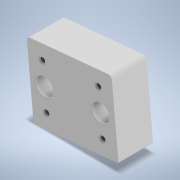
# Autodesk Inventor part: Head Spacer Plate
Saved by Autodesk Inventor 2020 (Build 240168000, 168)
## iProperties
Created: 2020-03-19
Part Number: Head Spacer Plate
Material: Generic
Document SubType Name: Modeling
Designer: DasNick
Density: 1 g/cm^3
Appearance: Default
Author: DasNick
Autodesk Inventor part; units mm, degrees
ref_plane "YZ Plane" through (0, 0, 0) normal (1, 0, 0) x (0, 1, 0)
ref_plane "XZ Plane" through (0, 0, 0) normal (0, 1, 0) x (-1, 0, 0)
ref_plane "XY Plane" through (0, 0, 0) normal (0, 0, 1) x (1, 0, 0)
sketch "Sketch1" plane through (0, 0, 0) normal (0, 0, 1) x (1, 0, 0)
  arc A0 (17.6188, 35.9553) -> (15.4359, 37.7539) centre (15.6281, 35.7632) ccw projected
  line L0 (15.4359, 37.7539) -> (-27.3652, 33.6227) projected
  arc A1 (-27.3652, 33.6227) -> (-29.1638, 31.4398) centre (-27.173, 31.6319) ccw projected
  line L1 (-29.1638, 31.4398) -> (-25.5552, -5.9466) projected
  arc A2 (-25.5552, -5.9466) -> (-25.0095, -6.3962) centre (-25.0575, -5.8985) ccw projected
  line L2 (-25.0095, -6.3962) -> (20.7777, -1.9768) projected
  arc A3 (20.7777, -1.9768) -> (21.2274, -1.4311) centre (20.7297, -1.4791) ccw projected
  line L3 (21.2274, -1.4311) -> (17.6188, 35.9553) projected
  circle A4 centre (-19.4703, 14.2799) radius 4.75 projected
  circle A5 centre (11.3863, 17.2582) radius 4.75 projected
  circle A6 centre (-18.3261, 2.3283) radius 1.25 projected
  circle A7 centre (10.2334, 29.2027) radius 1.25 projected
  circle A8 centre (-20.6232, 26.2244) radius 1.25 projected
  circle A9 centre (12.5491, 5.3084) radius 1.25 projected
  circle A10 centre (-18.3261, 2.3283) radius 1.5
  circle A11 centre (12.5491, 5.3084) radius 1.5
  circle A12 centre (10.2334, 29.2027) radius 1.5
  circle A13 centre (-20.6232, 26.2244) radius 1.5
  point P0 (0, 0)
  dimension "d0" = 3
  dimension "d1" = 3
  dimension "d3" = 3
  dimension "d6" = 3
  constraints: 4 centre point, 4 coincident
  measures "d0" diameter of A10
  measures "d1" diameter of A11
  measures "d3" diameter of A12
  measures "d6" diameter of A13
extrude "Extrusion1" add sketch "Sketch1" along normal blind 19.05 contours L3 A3 L2 A2 L1 A1 L0 A0
body "Solid1"
